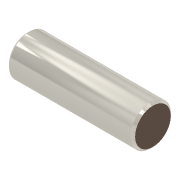
# Autodesk Inventor part: Axle Big
Saved by Autodesk Inventor 2022.2 (Build 262287010, 287A)
## iProperties
Created: 2022-12-22
Part Number: Axle Big
Material: Steel
Document SubType Name: Modeling
Designer: User
Density: 7.85 g/cm^3
Appearance: Gunmetal - Antique Polished
Author: User
Autodesk Inventor part; units mm, degrees
ref_plane "YZ Plane" through (0, 0, 0) normal (1, 0, 0) x (0, 1, 0)
ref_plane "XZ Plane" through (0, 0, 0) normal (0, 1, 0) x (-1, 0, 0)
ref_plane "XY Plane" through (0, 0, 0) normal (0, 0, 1) x (1, 0, 0)
sketch "Sketch1" plane through (0, 0, 0) normal (0, 0, 1) x (1, 0, 0)
  line L0 (-14, 4.5) -> (14, 4.5)
  line L1 (14, 4.5) -> (14, 0)
  line L2 (14, 0) -> (-14, 0)
  line L3 (-14, 0) -> (-14, 4.5)
  point P0 (0, 0)
  point P1 (0, 0)
  dimension "d0" = 9
  dimension "d1" = 28
  constraints: 8 end point, 2 parallel, 1 coincident, 1 horizontal, 1 midpoint, 1 perpendicular
  measures "d0" diameter of L0 L2
  measures "d1" distance of L0.start L0.end
revolve "Revolution1" add sketch "Sketch1" angle 360 about axis through (14, 0, 0) along (-1, 0, 0)
chamfer "Chamfer1" distance 0.5 angle 45 2 edges at (-14, -4.5, 0) (14, -4.5, 0)
body "Solid1"
